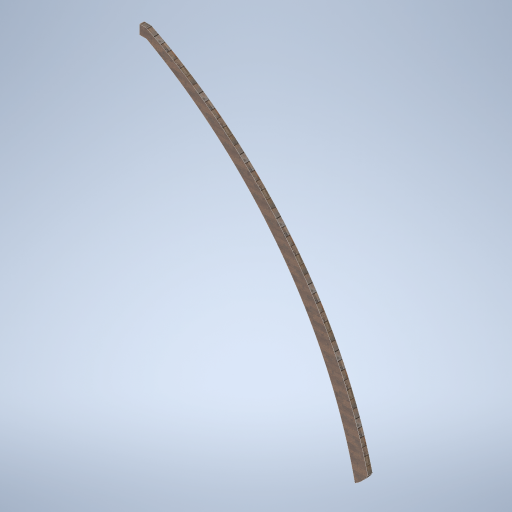
# Autodesk Inventor part: curve_beam_02
Saved by Autodesk Inventor 2024.2 (Build 282272000, 272)
## iProperties
Created: 2024-05-19
Part Number: curve_beam_02
Material: Wood (Maple)
Document SubType Name: Modeling
Designer: LOSTER_1
Density: 0.67 g/cm^3
Appearance: Natural Maple - Glossy Dark Tint
Author: LOSTER_1
Autodesk Inventor part; units mm, degrees
ref_plane "YZ Plane" through (0, 0, 0) normal (1, 0, 0) x (0, 1, 0)
ref_plane "XZ Plane" through (0, 0, 0) normal (0, 1, 0) x (-1, 0, 0)
ref_plane "XY Plane" through (0, 0, 0) normal (0, 0, 1) x (1, 0, 0)
sketch "Sketch1" plane through (0, 0, 0) normal (0, 0, 1) x (1, 0, 0)
  ellipse E0 centre (3487.9501, -1710.9027) end of major axis (3487.9501, -2510.9027) minor radius 800 (3896.5911, -2398.6618) -> (4173.8323, -2122.6862) ccw
  arc A0 (4173.8323, -2122.6862) -> (-553.1987, 3792.9367) centre (-4568.2524, -4261.8348) ccw
  arc A1 (3896.5911, -2398.6618) -> (-553.1987, 3592.9367) centre (-4903.3075, -4285.9308) ccw
  line L0 (-553.1987, 3792.9367) -> (-703.1987, 3792.9367)
  line L1 (-703.1987, 3792.9367) -> (-703.1987, 3592.9367)
  line L2 (-703.1987, 3592.9367) -> (-553.1987, 3592.9367)
  point P0 (0, 0)
  point P1 (3896.5911, -2398.6618)
  point P2 (4173.8323, -2122.6862)
  dimension "d0" = 9000
  dimension "d1" = 9000
  dimension "d2" = 150
  constraints: 6 end point, 4 point on circle, 2 centre point, 2 coincident, 2 perpendicular, 1 horizontal, 4 other
  measures "d0" radius of A0
  measures "d1" radius of A1
  measures "d2" distance of L0.start L0.end
extrude "Extrusion1" add sketch "Sketch1" along normal blind 100
body "Solid1"
